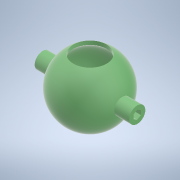
# Autodesk Inventor part: Dosificador
Saved by Autodesk Inventor 2020.1 (Build 241239000, 239)
## iProperties
Created: 2019-11-16
Part Number: Dosificador
Material: ABS Plastic
Document SubType Name: Modeling
Designer: Daniel
Density: 1.06 g/cm^3
Appearance: Smooth - Dark Forest Green
Author: Daniel
Autodesk Inventor part; units mm, degrees
ref_plane "XZ Plane" through (0, 0, 0) normal (0, 1, 0) x (-1, 0, 0)
ref_plane "XY Plane" through (0, 0, 0) normal (0, 0, 1) x (1, 0, 0)
sketch "Sketch8" plane through (0, 0, 0) normal (1, 0, 0) x (0, 1, 0)
  arc A0 (0, -31.02) -> (0, 31.02) centre (0, 0) ccw
  line L0 (0, 31.02) -> (0, -31.02)
  line L1 (0, -49.5025) -> (0, 42.4391) construction
  dimension "radio" = 31.02
  constraints: 4 end point, 4 point on line, 2 point on circle, 1 centre point, 1 coincident, 1 midpoint, 1 vertical
  measures "radio" radius of A0
revolve "Revolution2" add sketch "Sketch8" angle 360 about axis through (0, 0, -49.5025) along (0, 0, 1)
sketch "Sketch15" plane through (0, 0, 0) normal (0, 1, 0) x (-1, 0, 0)
  circle A0 centre (0, 0) radius 15.51
  dimension "d35" = 31.02
  constraints: 1 centre point, 1 coincident
  measures "d35" diameter of A0
extrude "Extrusion9" cut sketch "Sketch15" along normal up to surface
shell "Shell5" thickness 3 removed faces 2 at (0, 8.9547, 15.51) at (-6.3263, 0, 3.7266)
ref_plane "Work Plane6" through (44, 0, 0) normal (1, 0, 0) x (0, 1, 0)
sketch "Sketch13" plane through (44, 0, 0) normal (1, 0, 0) x (0, 1, 0)
  circle A0 centre (0, 0) radius 7.5
  dimension "d32" = 15
  constraints: 1 centre point, 1 coincident
  measures "d32" diameter of A0
extrude "Extrusion8" add sketch "Sketch13" against normal up to next
mirror "Mirror1" about plane through (0, 0, 0) normal (1, 0, 0) of "Extrusion8"
sketch "Sketch16" plane through (44, 0, 0) normal (1, 0, 0) x (0, 0, -1)
  circle A0 centre (0, 0) radius 7.5 projected
  circle A1 centre (0, 0) radius 4 construction
  line L0 (0, 4) -> (3.4641, 2)
  line L1 (3.4641, 2) -> (3.4641, -2)
  line L2 (3.4641, -2) -> (0, -4)
  line L3 (0, -4) -> (-3.4641, -2)
  line L4 (-3.4641, -2) -> (-3.4641, 2)
  line L5 (-3.4641, 2) -> (0, 4)
  dimension "d40" = 3.5
  constraints: 12 end point, 1 coincident, 1 vertical, 1 vertical alignment, 15 other
extrude "Extrusion10" cut sketch "Sketch16" against normal blind 10 contours L0 L1 L2 L3 L4 L5
equation "\"d35\" = radio"
body "Solid4"
